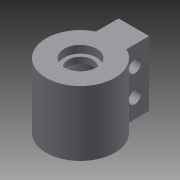
# Autodesk Inventor part: brush holder
Saved by Autodesk Inventor 2013 SP2 (Build 170200200, 200)
## iProperties
Created: 2017-05-15
Part Number: brush holder
Material: Generic
Document SubType Name: Modeling
Designer: Herman de Vries
Density: 1 g/cm^3
Author: Herman de Vries
Autodesk Inventor part; units mm, degrees
ref_plane "YZ Plane" through (0, 0, 0) normal (1, 0, 0) x (0, 1, 0)
ref_plane "XZ Plane" through (0, 0, 0) normal (0, 1, 0) x (-1, 0, 0)
ref_plane "XY Plane" through (0, 0, 0) normal (0, 0, 1) x (1, 0, 0)
sketch "Sketch1" plane through (0, 0, 0) normal (1, 0, 0) x (0, 1, 0)
  line L0 (0, 15) -> (2.5, 15) construction
  line L1 (0, 0) -> (9.4946, 0) construction
  arc A0 (9.4946, 0) -> (2.5, 15) centre (-10.0865, 0) ccw construction
  line L2 (0, 9.5) -> (0, 0) construction
  line L3 (9.4946, 0) -> (9, 0) construction
  line L4 (9, 0) -> (9, 15)
  line L5 (9, 15) -> (9, 15)
  line L6 (9, 15) -> (9, 17)
  line L7 (9, 17) -> (4.25, 17)
  line L8 (4.25, 17) -> (4.25, 15)
  line L9 (2.5, 15) -> (4.25, 15) construction
  line L10 (2.5, 15) -> (9.4946, 0) construction
  line L11 (3.25, 15) -> (3.25, 13.3916)
  line L12 (3.25, 15) -> (4.25, 15)
  line L13 (7.1631, 5) -> (7.1631, 0)
  line L14 (7.1631, 0) -> (9, 0)
  line L15 (7.1631, 5) -> (3.25, 13.3916)
  point P0 (2.25, 0)
  dimension "d2" = 15
  dimension "d12" = 2
  dimension "d14" = 0
  dimension "d16" = 2
  dimension "d17" = 4.25
  dimension "d35" = 115
  dimension "d36" = 9
  dimension "d37" = 2.5
  dimension "d39" = 1
  dimension "d40" = 5
  dimension "d41" = 7.1631
  dimension "d42" = 3.25
  dimension "d43" = 1.6084
  dimension "d44" = 8.3916
  constraints: 32 end point, 5 point on line, 4 collinear, 4 parallel, 4 perpendicular, 2 point on circle, 1 centre point, 1 horizontal, 1 line through centre, 1 vertical, 1 vertical alignment
  measures "d2" distance between parallel lines of L0 L1
  measures "d12" distance of L5.end L6.end
  measures "d14" distance of L4.end L5.end
  measures "d16" distance of L8.end L7.end
  measures "d17" distance between parallel lines of L2 L8
  measures "d35" angle of L10 L3
  measures "d36" distance from line of L4 L1.start
  measures "d37" distance from line of L2 L0.end
  measures "d39" distance between parallel lines of L8 L11
  measures "d40" distance of L13.start L13.end
  measures "d41" distance between parallel lines of L2 L13
  measures "d42" distance between parallel lines of L2 L11
  measures "d43" distance of L11.start L11.end
  measures "d44" vertical distance of L13.start L11.end
revolve "Revolution1" add sketch "Sketch1" angle 360 about axis through (0, 0, 9.5) along (0, 0, -1)
sketch "Sketch3" plane through (0, 0, 0) normal (1, 0, 0) x (0, 1, 0)
  line L0 (7.1631, 0) -> (14, 0)
  line L1 (14, 0) -> (14, 17)
  line L2 (14, 17) -> (7.1631, 17)
  line L3 (7.1631, 17) -> (7.1631, 0)
  line L4 (-7.1631, 0) -> (7.1631, 0) construction
  line L5 (-9, 17) -> (9, 17) construction
  point P0 (0, 0)
  dimension "d28" = 14
  constraints: 8 end point, 2 parallel, 1 horizontal, 1 perpendicular, 1 point on line
  measures "d28" distance from line of L1 point (0, 0)
extrude "Extrusion1" add sketch "Sketch3" along normal mid plane 8
sketch "Sketch4" plane through (-4, 0, 0) normal (-1, 0, 0) x (0, 0, 1)
  circle A0 centre (5, 10.25) radius 1.6
  circle A1 centre (12, 10.25) radius 1.6
  line L0 (5, 10.25) -> (12, 10.25) construction
  line L1 (17, 14) -> (0, 14) construction
  point P0 (0, 0)
  point P1 (17, 10.25)
  point P2 (8.5, 10.25)
  point P3 (8.5, 14)
  dimension "d29" = 3.2
  dimension "d30" = 3.2
  dimension "d31" = 7
  dimension "d34" = 3.75
  constraints: 2 centre point, 2 end point, 2 horizontal alignment, 2 midpoint, 1 horizontal, 1 vertical alignment
  measures "d29" diameter of A0
  measures "d30" diameter of A1
  measures "d31" distance of L0.start L0.end
  measures "d34" distance between parallel lines of L0 L1
extrude "Extrusion2" cut sketch "Sketch4" against normal blind 10
body "Solid1"
